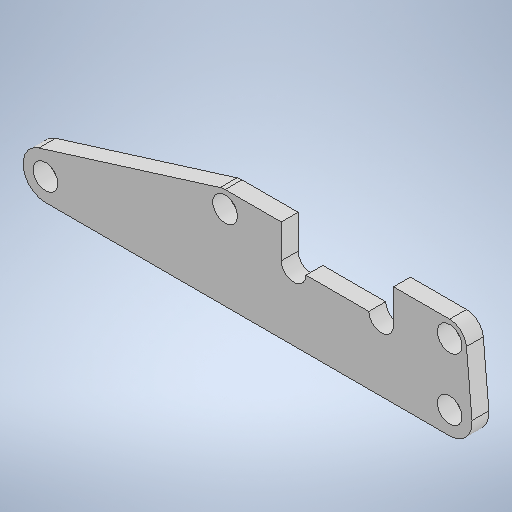
# Autodesk Inventor part: kosiyosetuzoku
Saved by Autodesk Inventor 2025.1 (Build 291241000, 241)
## iProperties
Created: 2024-08-31
Part Number: kosiyosetuzoku
Material: 一般
Document SubType Name: Modeling
Designer: right
Density: 1 g/cm^3
Appearance: 既定
Author: right
Autodesk Inventor part; units mm, degrees
ref_plane "YZ Plane" through (0, 0, 0) normal (1, 0, 0) x (0, 1, 0)
ref_plane "XZ Plane" through (0, 0, 0) normal (0, 1, 0) x (-1, 0, 0)
ref_plane "XY Plane" through (0, 0, 0) normal (0, 0, 1) x (1, 0, 0)
sketch "スケッチ1" plane through (0, 0, 0) normal (0, 0, 1) x (1, 0, 0)
  circle A0 centre (-18, 0) radius 1.1
  circle A1 centre (18, 0) radius 1.1
  circle A2 centre (-18, 0) radius 2
  circle A3 centre (18, 0) radius 2
  line L0 (3, 7) -> (13, 7)
  line L1 (13, 7) -> (13, 4)
  line L2 (13, 4) -> (3, 4)
  line L3 (3, 4) -> (3, 7)
  circle A4 centre (4.1, 4) radius 1.1
  line L4 (8, 7) -> (8, 3.6941) construction
  circle A5 centre (11.9, 4) radius 1.1
  circle A6 centre (18, 5.5) radius 1.1
  circle A7 centre (-2, 5.5) radius 1.1
  circle A8 centre (-2, 5.5) radius 1.5
  circle A9 centre (18, 5.5) radius 1.5
  line L5 (-18.594, 1.9098) -> (-2.4455, 6.9323)
  line L6 (-2, 7) -> (3, 7)
  line L7 (3, 7) -> (3, 7)
  line L8 (19.4938, 5.6364) -> (19.9917, 0.1818)
  line L9 (-18, -2) -> (18, -2)
  line L10 (18, 7) -> (13, 7)
  line L11 (13, 7) -> (13, 7)
  point P0 (0, 0)
  point P1 (13, 5.5)
  point P2 (10.8, 4)
  point P3 (5.2, 4)
  dimension "d0" = 2.2
  dimension "d1" = 2.2
  dimension "d2" = 36
  dimension "d3" = 18
  dimension "d4" = 4
  dimension "d5" = 4
  dimension "d6" = 3
  dimension "d7" = 10
  dimension "d8" = 2.2
  dimension "d9" = 2.2
  dimension "d10" = 5
  dimension "d11" = 3
  dimension "d12" = 3
  dimension "d13" = 4
  constraints: 24 end point, 10 centre point, 9 tangent, 8 point on circle, 4 coincident, 3 horizontal, 3 horizontal alignment, 3 perpendicular, 2 midpoint, 2 parallel, 2 symmetric about line, 1 point on line, 1 vertical, 1 vertical alignment, 2 other
  measures "d0" diameter of A0
  measures "d1" diameter of A1
  measures "d2" distance of A1.centre A0.centre
  measures "d3" distance of point (0, 0) A1.centre
  measures "d4" diameter of A2
  measures "d5" diameter of A3
  measures "d6" distance between parallel lines of L2 L0
  measures "d7" distance of L0.start L0.end
  measures "d8" diameter of A4
  measures "d9" diameter of A6
  measures "d10" distance from line of L1 A6.centre
  measures "d11" diameter of A8
  measures "d12" diameter of A9
  measures "d13" vertical distance of A1.centre A5.centre
extrude "押し出し1" add sketch "スケッチ1" along normal blind 1.5 contours A2 | A2 L5 A8 L6 L3 A4 L2 A5 L1 L10 A9 L8 A3 L9 | A8 | A3 | A9
equation "\"d3\" = 0.5 * d2"
equation "\"d12\" = d11"
